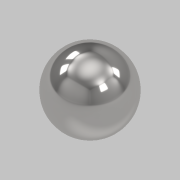
# Autodesk Inventor part: 볼
Saved by Autodesk Inventor 2020 (Build 240168000, 168)
## iProperties
Created: 2020-06-01
Part Number: 볼
Material: 일반
Document SubType Name: Modeling
Designer: Miji
Density: 1 g/cm^3
Appearance: 강철 - 연마
Author: Miji
Autodesk Inventor part; units mm, degrees
ref_plane "YZ Plane" through (0, 0, 0) normal (1, 0, 0) x (0, 1, 0)
ref_plane "XZ Plane" through (0, 0, 0) normal (0, 1, 0) x (-1, 0, 0)
ref_plane "XY Plane" through (0, 0, 0) normal (0, 0, 1) x (1, 0, 0)
sketch "스케치1" plane through (0, 0, 0) normal (1, 0, 0) x (0, 1, 0)
  line L0 (0, 0) -> (16, 0)
  arc A0 (0, 0) -> (16, 0) centre (8, 0) ccw
  dimension "d0" = 16
  dimension "d0" = 16
  constraints: 2 end point, 2 point on circle, 1 centre point, 1 horizontal, 1 midpoint
  measures "d0" distance of L0.start L0.end
revolve "회전1" add sketch "스케치1" angle 360 about axis through (0, 0, 0) along (0, 1, 0)
